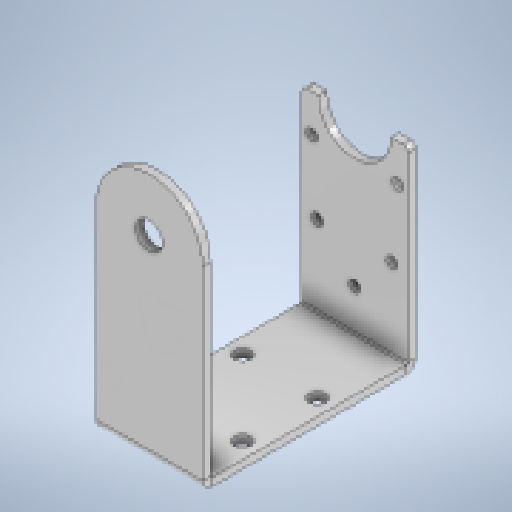
# Autodesk Inventor part: axis_9_bottom_frame
Saved by Autodesk Inventor 2026.1 (Build 301233000, 233)
## iProperties
Created: 2025-05-04
Part Number: axis_9_bottom_frame
Material: Aluminum 6061-AHC
Document SubType Name: Sheet Metal
Designer: User
Density: 2.7 g/cm^3
Sheet Metal Rule: Default_mm
Appearance: Aluminum - Dark
Flat Pattern Width: 2 cm
Flat Pattern Length: 11.6859 cm
Flat Pattern Area: 23.3717 cm^2
Sheet Metal Width: 20.000 mm
Sheet Metal Length: 116.859 mm
Sheet Metal Area: 2337.171 mm^2
Author: User
Autodesk Inventor part; units mm, degrees
ref_plane "YZ Plane" through (0, 0, 0) normal (1, 0, 0) x (0, 1, 0)
ref_plane "XZ Plane" through (0, 0, 0) normal (0, 1, 0) x (-1, 0, 0)
ref_plane "XY Plane" through (0, 0, 0) normal (0, 0, 1) x (1, 0, 0)
sketch "Sketch1" plane through (0, 0, 0) normal (0, 1, 0) x (-1, 0, 0)
  line L0 (10, -17.5) -> (-10, -17.5)
  line L1 (-10, -17.5) -> (-10, 18.5)
  line L2 (-10, 18.5) -> (10, 18.5)
  line L3 (10, 18.5) -> (10, -17.5)
  point P0 (0, 0)
  dimension "d0" = 20
  dimension "d1" = 36
  dimension "d2" = 17.5
  dimension "d3" = 10
  constraints: 8 end point, 2 parallel, 1 horizontal, 1 perpendicular
  measures "d0" distance of L0.start L0.end
  measures "d1" distance of L0.end L1.end
  measures "d2" distance from line of L0 point (0, 0)
  measures "d3" distance from line of point (0, 0) L3
extrude "Plate1" add sketch "Sketch1" along normal blind 1.5
sketch "Sketch2" plane through (-10, 0, -19) normal (0, 0, 1) x (1, 0, 0)
  line L0 (20, 0) -> (0, 0)
  line L1 (0, 0) -> (0, 46.6)
  line L2 (0, 46.6) -> (20, 46.6)
  line L3 (20, 46.6) -> (20, 0)
  constraints: 8 end point
edge flange "Flange1" height 46.6 angle 90 thickness 1.5 bend radius 0.31 thickness toward (0, 0, 1) relief tear relief width 1.5 relief depth 0.75 edges at (0, 1.5, -17.5) wall of the first edge with corners at (10, 0, -19) (-10, 0, -19) (-10, 46.6, -19) (10, 46.6, -19)
bend "Bend1"
corner "Corner1"
sketch "Sketch3" plane through (10, 0, 20) normal (0, 0, -1) x (-1, 0, 0)
  line L0 (20, 0) -> (0, 0)
  line L1 (0, 0) -> (0, 46.6)
  line L2 (0, 46.6) -> (20, 46.6)
  line L3 (20, 46.6) -> (20, 0)
  constraints: 8 end point
edge flange "Flange2" height 46.6 angle 90 thickness 1.5 bend radius 0.31 thickness toward (0, 0, -1) relief tear relief width 1.5 relief depth 0.75 edges at (0, 1.5, 18.5) wall of the first edge with corners at (-10, 0, 20) (10, 0, 20) (10, 46.6, 20) (-10, 46.6, 20)
bend "Bend2"
corner "Corner2"
sketch "Sketch4" plane through (-10, 46.6, 20) normal (0, 0, 1) x (1, 0, 0)
  circle A0 centre (10, -10) radius 10
  line L0 (0, 0) -> (20, 0) projected
  line L1 (0, 0) -> (20, 0)
  line L2 (20, 0) -> (20, -10)
  line L3 (20, -10) -> (0, -10)
  line L4 (0, -10) -> (0, 0)
  line L5 (0, -44.79) -> (0, 0) projected
  point P0 (10, -46.6)
  point P1 (10, -10)
  point P2 (20, 0)
  point P3 (10, 0)
  point P4 (0, -10)
  point P5 (8.5893, 0)
  point P6 (0, -10)
  dimension "d26" = 20
  dimension "d25" = 10
  dimension "d27" = 10
  dimension "d28" = 10
  constraints: 8 end point, 2 parallel, 1 horizontal, 1 midpoint, 1 perpendicular, 3 other
  measures "d25" distance from line of L0 point (10, -10)
  measures "d27" distance from line of point (10, -10) L2
  measures "d28" distance from line of L5 point (10, -10)
extrude "Extrusion1" cut sketch "Sketch4" against normal blind 10 contours L4 L0 A0 | A0 L0 L2
sketch "Sketch5" plane through (10, 46.6, -19) normal (0, 0, -1) x (-1, 0, 0)
  arc A0 (20, -10) -> (0, -10) centre (10, -10) ccw projected
  point P0 (10, -46.6)
hole "Hole1" at (0, 36.6, -19) direction (0, 0, 1) diameter 13.5 depth 1.5
sketch "Sketch6" plane through (10, 46.6, -19) normal (0, 0, -1) x (-1, 0, 0)
  circle A0 centre (10, -10) radius 6.75 projected
  line L0 (0, 0) -> (20, 0) projected
  line L1 (0, -44.79) -> (0, 0) projected
  line L2 (24, 0) -> (-4, 0)
  line L3 (-4, 0) -> (-4, -9.9)
  line L4 (-4, -9.9) -> (24, -9.9)
  line L5 (24, -9.9) -> (24, 0)
  point P0 (10, -46.6)
  point P1 (20, 0)
  point P2 (6.005, 0)
  point P3 (13.995, 0)
  dimension "d38" = 9.9
  dimension "d39" = 4
  dimension "d40" = 28
  constraints: 8 end point, 2 parallel, 1 horizontal, 1 perpendicular, 1 point on line, 1 other
  measures "d38" distance of L2.end L3.end
  measures "d39" distance between parallel lines of L1 L3
  measures "d40" distance between parallel lines of L5 L3
extrude "Extrusion2" cut sketch "Sketch6" against normal blind 10 contours L4 A0 | A0 L4 L1 L0 L2 L5 | L4 L3 L2 L1 picked at (7.8223, -9.3675)
fillet "Fillet1" radius 1 2 edges at (-10, 36.7, -18.25) (10, 36.7, -18.25)
sketch "Sketch7" plane through (-10, 1.81, 20) normal (0, 0, 1) x (1, 0, 0)
  arc A0 (20, 34.79) -> (0, 34.79) centre (10, 34.79) ccw projected
  point P0 (10, -1.81)
hole "Hole2" at (0, 36.6, 20) direction (0, 0, -1) diameter 5.1 depth 1.5 clearance for "Hex Head Bolt" size "M5" standard "Ansi Metric M Profile"
sketch "Sketch8" plane through (0, 0, 0) normal (0, -1, 0) x (1, 0, 0)
  line L0 (2.55, 18.5) -> (-2.55, 18.5) projected
  line L1 (-10, 18.5) -> (10, 18.5) projected
  line L2 (10, 18.5) -> (-10, 18.5) projected
  line L3 (10, 18.19) -> (-10, 18.19) projected
  line L4 (-10, -17.19) -> (-10, 18.19) projected
  line L5 (-10, -17.19) -> (10, -17.19) projected
  line L6 (10, 18.19) -> (10, -17.19) projected
  point P0 (0, 0)
  point P1 (7, 9.5)
  point P2 (7, -4.5)
  point P3 (-7, 9.5)
  point P4 (-7, -4.5)
  dimension "d51" = 9
  dimension "d52" = 3
  dimension "d55" = 14
  dimension "d58" = 14
  constraints: 1 horizontal, 1 vertical, 3 other
  measures "d51" distance from line of L1 point (7, 9.5)
  measures "d52" distance from line of L6 point (7, 9.5)
  measures "d55" distance of point (7, 9.5) point (7, -4.5)
  measures "d58" distance of point (7, 9.5) point (-7, 9.5)
hole "Hole3" at (7, 0, 9.5) at (7, 0, -4.5) at (-7, 0, 9.5) at (-7, 0, -4.5) direction (0, 1, 0) diameter 3 depth 1.5
hole "Hole5" at (-8, 29.7, -17.5) at (8, 29.7, -17.5) at (7, 16.48, -17.5) at (-7, 16.48, -17.5) at (0, 9.18, -17.5) direction (0, 0, -1) diameter 2.1 depth 1.5
sketch "Sketch11" plane through (-10, 1.81, 20) normal (0, 0, 1) x (1, 0, 0)
  circle A0 centre (10, 7.37) radius 1.1
  point P0 (10, -1.81)
  constraints: 1 centre point, 2 other
hole "Hole6" at (0, 9.18, 20) direction (0, 0, -1) diameter 3 depth 1.5
equation "\"d66\" = Thickness"
equation "\"d80\" = Thickness"
equation "\"d49\" = Thickness"
equation "\"d4\" = Thickness"
equation "\"d15\" = BendReliefWidth"
equation "\"d16\" = BendReliefDepth"
equation "\"d17\" = MinimumRemnant"
equation "\"d18\" = TransitionRadius"
equation "\"d21\" = BendRadius"
equation "\"d22\" = CornerReliefSize"
equation "\"d23\" = GapSize"
equation "\"d24\" = JacobiRadiusSize"
equation "\"d36\" = Thickness"
equation "\"d5\" = BendReliefWidth"
equation "\"d6\" = BendReliefDepth"
equation "\"d7\" = MinimumRemnant"
equation "\"d8\" = TransitionRadius"
equation "\"d11\" = BendRadius"
equation "\"d12\" = CornerReliefSize"
equation "\"d13\" = GapSize"
equation "\"d14\" = JacobiRadiusSize"
equation "\"d87\" = Thickness"
equation "\"BendReliefWidth\" = Thickness"
equation "\"BendReliefDepth\" = 0.5 * Thickness"
equation "\"CornerReliefSize\" = 4 * Thickness"
equation "\"MinimumRemnant\" = 2 * Thickness"
equation "\"TransitionRadius\" = BendRadius"
equation "\"JacobiRadiusSize\" = BendRadius"
equation "\"GapSize\" = Thickness"
equation "\"Thickness\" = 1.5"
equation "\"BendRadius\" = 0.31"
body "Solid1"
